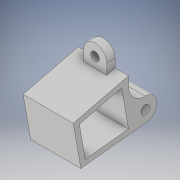
# Autodesk Inventor part: Camera Mount v2
Saved by Autodesk Inventor 2017 SP1 (Build 210196100, 196)
## iProperties
Created: 2016-10-03
Part Number: Camera Mount v2
Material: Generic
Document SubType Name: Modeling
Designer: Haden
Density: 1 g/cm^3
Appearance: Default
Author: Haden
Autodesk Inventor part; units mm, degrees
ref_plane "YZ Plane" through (0, 0, 0) normal (1, 0, 0) x (0, 1, 0)
ref_plane "XZ Plane" through (0, 0, 0) normal (0, 1, 0) x (-1, 0, 0)
ref_plane "XY Plane" through (0, 0, 0) normal (0, 0, 1) x (1, 0, 0)
sketch "Sketch1" plane through (0, 0, 0) normal (1, 0, 0) x (0, 1, 0)
  line L0 (-13.2874, 37.3275) -> (-38.5145, 32.8793)
  line L1 (-38.5145, 32.8793) -> (-34.9427, 0)
  line L2 (-34.9427, 0) -> (-5.3985, 5.2094)
  line L3 (-5.3985, 5.2094) -> (-13.2874, 37.3275)
  line L4 (0, 0) -> (-10.2957, 41.9167)
  line L5 (-10.2957, 41.9167) -> (-42.8954, 36.1685)
  line L6 (-42.8954, 36.1685) -> (-37.4823, -13.6601)
  line L7 (-19.7543, -12.7) -> (-19.7543, 0)
  arc A0 (-37.4823, -13.6601) -> (-19.7543, -12.7) centre (-28.6443, -12.7) ccw
  circle A1 centre (-28.6443, -12.7) radius 3.302
  line L8 (0, 0) -> (-19.7543, 0)
  dimension "d8" = 33
  dimension "d9" = 86.2
  dimension "d10" = 86.2
  dimension "d11" = 30
  dimension "d13" = 4
  dimension "d14" = 4
  dimension "d15" = 4
  dimension "d22" = 8.89
  dimension "d23" = 6.604
  dimension "d24" = 12.7
  dimension "d25" = 100
  constraints: 18 end point, 4 parallel, 3 point on circle, 2 centre point, 2 coincident, 2 point on line, 2 tangent, 1 horizontal, 1 vertical
  measures "d8" distance between parallel lines of L2 L0
  measures "d9" angle of L2 L3
  measures "d10" angle of L2 L1
  measures "d11" distance of L1.end L2.end
  measures "d13" distance between parallel lines of L5 L0
  measures "d14" distance between parallel lines of L4 L3
  measures "d15" distance between parallel lines of L1 L6
  measures "d22" radius of A0
  measures "d23" diameter of A1
  measures "d24" vertical distance of A0.centre point (0, 0)
  measures "d25" angle of L2 L7
extrude "Extrusion2" add sketch "Sketch1" along normal blind 38.1
fillet "Fillet2" radius 12.7 1 edges at (19.05, -19.7543, 0)
ref_plane "Work Plane1" through (38.1, 0, 6.35) normal (0, 0, -1) x (-1, 0, 0)
sketch "Sketch2" plane through (38.1, 0, 6.35) normal (0, 0, -1) x (-1, 0, 0)
  line L0 (27.94, -1.5597) -> (27.94, 6.35)
  line L1 (10.16, 6.35) -> (10.16, -1.5597)
  arc A0 (27.94, 6.35) -> (10.16, 6.35) centre (19.05, 6.35) ccw
  circle A1 centre (19.05, 6.35) radius 3.302
  line L2 (38.1, -39.6561) -> (0, -39.6561) projected
  line L3 (0, -39.6561) -> (0, -35.6325) projected
  line L4 (0, -35.6325) -> (38.1, -35.6325) projected
  line L5 (38.1, -35.6325) -> (38.1, -39.6561) projected
  line L6 (0, -1.5597) -> (38.1, -1.5597) projected
  line L7 (38.1, -1.5597) -> (38.1, -5.6786) projected
  line L8 (38.1, -5.6786) -> (0, -5.6786) projected
  line L9 (0, -5.6786) -> (0, -1.5597) projected
  line L10 (38.1, 0) -> (0, 0) projected
  point P0 (19.05, -1.5597)
  dimension "d31" = 6.604
  dimension "d32" = 8.89
  dimension "d33" = 6.35
  constraints: 4 end point, 2 centre point, 2 point on circle, 2 point on line, 2 tangent, 2 vertical, 1 concentric, 1 midpoint, 1 vertical alignment
  measures "d31" diameter of A1
  measures "d32" radius of A0
  measures "d33" distance from line of L10 A0.centre
extrude "Extrusion3" add sketch "Sketch2" along normal up to surface (6.35 mm away) contours L6 L1 L10 L0 | L10 L1 A0 L0
body "Solid2"
